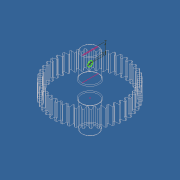
# Autodesk Inventor part: ENGR.RETA MOVIDA
Saved by Autodesk Inventor 2012 SP1 (Build 160190100, 190)
## iProperties
Created: 2012-07-24
Part Number: ENGR.RETA MOVIDA
Material: Carbon Steel
Document SubType Name: Modeling
Designer: bruno.silveira
Mass: 144.637 g
Surface Area: 55.8418 cm^2
Volume: 18.3783 cm^3
Density: 7.87 g/cm^3
Author: bruno.silveira
Autodesk Inventor part; units mm, degrees
ref_plane "YZ Plane" through (0, 0, 0) normal (1, 0, 0) x (0, 1, 0)
ref_plane "XZ Plane" through (0, 0, 0) normal (0, 1, 0) x (-1, 0, 0)
ref_plane "XY Plane" through (0, 0, 0) normal (0, 0, 1) x (1, 0, 0)
sketch "Sketch1" plane through (0, 0, 0) normal (0, 0, 1) x (1, 0, 0)
  circle A0 centre (0, 0) radius 22.5
  dimension "d0" = 45
  constraints: 1 centre point, 1 coincident
  measures "d0" diameter of A0
extrude "Extrusion1" add sketch "Sketch1" along normal blind 10
sketch "Sketch2" plane through (0, 0, 10) normal (0, 0, 1) x (1, 0, 0)
  circle A0 centre (0, 0) radius 22.5 projected
  circle A1 centre (0, 0) radius 5
  dimension "d3" = 10
  constraints: 1 centre point, 1 coincident
  measures "d3" diameter of A1
extrude "Extrusion2" add sketch "Sketch2" along normal blind 15 contours A1
sketch "Sketch3" plane through (0, 0, 0) normal (0, 0, -1) x (-1, 0, 0)
  circle A0 centre (0, 0) radius 22.5 projected
  circle A1 centre (0, 0) radius 5
  dimension "d6" = 10
  constraints: 1 centre point, 1 coincident
  measures "d6" diameter of A1
extrude "Extrusion3" add sketch "Sketch3" along normal blind 16.5 contours A1
spur gear teeth "Spur Gear1" teeth 43 pitch diameter 43 tip diameter 44.9141 root diameter 40.5 face width 10 trims to tip circle yes start plane through (0, 0, 10) normal (0, 0, 1) x (1, 0, 0)
chamfer "Chamfer1" distance 0.5 angle 45 2 edges at (-5, 0, 25) (5, 0, -16.5)
fillet "Fillet1" radius 0.5 2 edges at (5, 0, 0) (-5, 0, 10)
sketch "Sketch4" plane through (0, 0, 0) normal (1, 0, 0) x (0, 1, 0)
  line L0 (5, 24.5) -> (-5, 24.5) projected
  line L1 (-5, 10.5) -> (5, 10.5) projected
  circle A0 centre (0, 18) radius 1.5
  line L2 (-4.5, 25) -> (4.5, 25) projected
  point P0 (0, 0)
  dimension "d13" = 3
  dimension "d14" = 7
  constraints: 1 centre point
  measures "d13" diameter of A0
  measures "d14" distance from line of L2 A0.centre
extrude "Extrusion4" cut sketch "Sketch4" along normal mid plane 12
body "Solid1"
